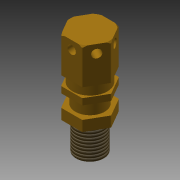
# Autodesk Inventor part: fc18-055
Saved by Autodesk Inventor 2018 (Build 220112000, 112)
## iProperties
Category: Pneumatics
Company: Autodesk, Inc.
Shininess: 64.0
Length Units: 11269
Angle Units: 11279
Time Units: 11290
Mass Units: 11283
Length Display Precision: 3
Angle Display Precision: 2
Compacted: True
Part Number: fc18-055
Document SubType Name: Modeling
Created: 2017-11-24
Manufacturer: Standard
Standards Organization: Custom
Material: Brass, Soft Yellow
Catalog Web Link: http://cdn.norgren.com/pdf/16-004.pdf
Description: Pressure Relief Valve
Vendor: Norgren
Mass: 77.0566 g
Surface Area: 45.3009 cm^2
Volume: 9.09759 cm^3
Density: 8.47 g/cm^3
Project: FIRST
Appearance: Brass - Satin
Stock Number: 16-004-011
Density: 0.0
Volumn: 0.0
Area: 0.0
PropertySet Name: Model Information
Control State: 0
Master: False
Checked Out: False
Title: Pressure Relief Valve
Author: Autodesk, Inc.
Keywords: FIRST Choice
Autodesk Inventor part; units mm, degrees
ref_plane "YZ Plane" through (0, 0, 0) normal (1, 0, 0) x (0, 1, 0)
ref_plane "XZ Plane" through (0, 0, 0) normal (0, 1, 0) x (-1, 0, 0)
ref_plane "XY Plane" through (0, 0, 0) normal (0, 0, 1) x (1, 0, 0)
sketch "Sketch1" plane through (0, 0, 0) normal (0, 0, 1) x (1, 0, 0)
  line L0 (5.0518, 8.75) -> (10.1036, 0)
  line L1 (10.1036, 0) -> (5.0518, -8.75)
  line L2 (5.0518, -8.75) -> (-5.0518, -8.75)
  line L3 (-5.0518, -8.75) -> (-10.1036, 0)
  line L4 (-10.1036, 0) -> (-5.0518, 8.75)
  line L5 (-5.0518, 8.75) -> (5.0518, 8.75)
  point P0 (0, 0)
  point P1 (0, 0)
  dimension "d0" = 17.5
  constraints: 12 end point, 1 coincident, 1 horizontal, 11 other
  measures "d0" distance between parallel lines of L2 L5
extrude "Extrusion1" add sketch "Sketch1" against normal blind 17
sketch "Sketch2" plane through (0, 0, -17) normal (0, 0, -1) x (-1, 0, 0)
  line L0 (-5.0518, 8.75) -> (5.0518, 8.75) projected
  line L1 (-10.1036, 0) -> (-5.0518, 8.75) projected
  line L2 (-5.0518, -8.75) -> (-10.1036, 0) projected
  line L3 (5.0518, -8.75) -> (-5.0518, -8.75) projected
  line L4 (10.1036, 0) -> (5.0518, -8.75) projected
  line L5 (5.0518, 8.75) -> (10.1036, 0) projected
  line L6 (-5.0518, 8.75) -> (5.0518, 8.75) projected
  circle A0 centre (0, 0) radius 8.25
  dimension "d3" = 16.5
  constraints: 1 centre point
  measures "d3" diameter of A0
extrude "Extrusion2" add sketch "Sketch2" along normal blind 4.5 contours A0
sketch "Sketch3" plane through (0, 0, -21.5) normal (0, 0, -1) x (-1, 0, 0)
  circle A0 centre (0, 0) radius 8.25 projected
  line L0 (-5.0518, 8.75) -> (5.0518, 8.75) projected
  line L1 (-10.1036, 0) -> (-5.0518, 8.75) projected
  line L2 (-5.0518, -8.75) -> (-10.1036, 0) projected
  line L3 (5.0518, -8.75) -> (-5.0518, -8.75) projected
  line L4 (10.1036, 0) -> (5.0518, -8.75) projected
  line L5 (5.0518, 8.75) -> (10.1036, 0) projected
extrude "Extrusion3" add sketch "Sketch3" along normal blind 3 contours A0 | L0 L5 L4 L3 L2 L1
sketch "Sketch4" plane through (0, 0, -24.5) normal (0, 0, -1) x (-1, 0, 0)
  line L0 (5.0518, 8.75) -> (10.1036, 0) projected
  line L1 (-5.0518, 8.75) -> (5.0518, 8.75) projected
  line L2 (-10.1036, 0) -> (-5.0518, 8.75) projected
  line L3 (-5.0518, -8.75) -> (-10.1036, 0) projected
  line L4 (5.0518, -8.75) -> (-5.0518, -8.75) projected
  line L5 (10.1036, 0) -> (5.0518, -8.75) projected
  circle A0 centre (0, 0) radius 7
  dimension "d8" = 14
  constraints: 1 centre point
  measures "d8" diameter of A0
extrude "Extrusion4" add sketch "Sketch4" along normal blind 6 contours A0
sketch "Sketch5" plane through (0, 0, -30.5) normal (0, 0, -1) x (-1, 0, 0)
  circle A0 centre (0, 0) radius 7 projected
  line L0 (5.0518, 8.75) -> (10.1036, 0) projected
  line L1 (-5.0518, 8.75) -> (5.0518, 8.75) projected
  line L2 (-10.1036, 0) -> (-5.0518, 8.75) projected
  line L3 (-5.0518, -8.75) -> (-10.1036, 0) projected
  line L4 (5.0518, -8.75) -> (-5.0518, -8.75) projected
  line L5 (10.1036, 0) -> (5.0518, -8.75) projected
extrude "Extrusion5" add sketch "Sketch5" along normal blind 5 contours A0 | L0 L5 L4 L3 L2 L1
sketch "Sketch6" plane through (0, 0, -35.5) normal (0, 0, -1) x (-1, 0, 0)
  line L0 (10.1036, 0) -> (5.0518, -8.75) projected
  line L1 (5.0518, 8.75) -> (10.1036, 0) projected
  line L2 (-5.0518, 8.75) -> (5.0518, 8.75) projected
  line L3 (-10.1036, 0) -> (-5.0518, 8.75) projected
  line L4 (-5.0518, -8.75) -> (-10.1036, 0) projected
  line L5 (5.0518, -8.75) -> (-5.0518, -8.75) projected
  circle A0 centre (0, 0) radius 6.625
  dimension "d13" = 13.25
  constraints: 1 centre point
  measures "d13" diameter of A0
extrude "Extrusion6" add sketch "Sketch6" along normal blind 14.5 contours A0
sketch "Sketch7" plane through (0, 0, -50) normal (0, 0, -1) x (-1, 0, 0)
  circle A0 centre (0, 0) radius 6.625 projected
  circle A1 centre (0, 0) radius 2.5
  dimension "d16" = 5
  constraints: 1 centre point, 1 coincident
  measures "d16" diameter of A1
extrude "Extrusion7" cut sketch "Sketch7" against normal blind 47.5 contours A1
sketch "Sketch8" plane through (-5.0518, 8.75, 0) normal (0, 1, 0) x (1, 0, 0)
  line L0 (10.1036, 17) -> (0, 17) projected
  line L1 (0, 0) -> (0, 17) projected
  line L2 (0, 0) -> (10.1036, 0) projected
  line L3 (10.1036, 0) -> (10.1036, 17) projected
  circle A0 centre (5.0518, 4) radius 2
  dimension "d19" = 4
  dimension "d20" = 4
  constraints: 1 centre point
  measures "d19" diameter of A0
  measures "d20" distance from line of L2 A0.centre
extrude "Extrusion8" cut sketch "Sketch8" against normal blind 40.25 contours A0
pattern_circular "Circular Pattern1" count 3 over 360 about axis through (0, 0, -17) along (0, 0, -1) of "Extrusion8"
thread "Thread1" size "1/4" designation "1/4 - 18 NPT" standard "NPT" full length
fillet "Fillet1" radius 0.5 18 edges at (-5.0518, -8.75, -8.5) (5.0518, -8.75, -8.5) (10.1036, 0, -8.5) (5.0518, 8.75, -8.5) (-5.0518, 8.75, -8.5) (-10.1036, 0, -8.5) (-5.0518, -8.75, -23) (5.0518, -8.75, -23) (10.1036, 0, -23) (5.0518, 8.75, -23) (5.0518, 8.75, -33) (10.1036, 0, -33) (5.0518, -8.75, -33) (-5.0518, -8.75, -33) (-10.1036, 0, -23) (-5.0518, 8.75, -23) (-5.0518, 8.75, -33) (-10.1036, 0, -33)
sketch "Sketch10" plane through (0, 0, 0) normal (0, 1, 0) x (-1, 0, 0)
  line L0 (10.0263, 0) -> (10.0263, -17) projected
  line L1 (9.9593, 0) -> (5.1962, 0) projected
  line L2 (9.9593, -17) -> (9.9593, -17) projected
  line L3 (9.9593, -17) -> (9.9593, 0) projected
  line L4 (9.9593, 0) -> (9.9593, 0) projected
  line L5 (9.9593, 0) -> (9.9593, -17) projected
  ellipse E0 centre (7.5777, -4) end of major axis (7.5777, -2) minor radius 1 projected
  line L6 (9.9593, 0) -> (9.9593, -17) projected
  line L7 (9.9593, 0) -> (5.1962, 0) projected
  line L8 (5.1962, -17) -> (5.1962, 0) projected
  line L9 (5.1962, -17) -> (9.9593, -17) projected
  line L10 (10.0263, -0.7071) -> (9.3192, 0)
  line L11 (9.3192, 0) -> (10.0263, 0)
  line L12 (10.0263, -0.7071) -> (10.0263, 0)
  line L13 (0, -20.4) -> (0, 3.4) projected
  dimension "d32" = 45
  dimension "d33" = 1
  constraints: 6 end point, 2 point on line, 1 parallel, 1 perpendicular, 1 other
  measures "d32" angle of L0 L10
  measures "d33" distance of L10.start L10.end
revolve "Revolution2" cut sketch "Sketch10" angle 360 about axis through (0, 0, -10) along (0, 0, 1) contours L0 L10 L3 L11 | L3 L10 L1
equation "\"d20\" = d19"
body "Solid1"
